Autodesk Fusion 360 part; units mm, degrees
(part 2 of 2)
  measures "d135" diameter of A4
extrude "Extrude12" add sketch "Lid (main and holes)" along normal blind 2 separate body makes body 2
extrude "Extrude13" add sketch "Lid (main and holes)" against normal blind 44 contours L2 L7 L8 L9 L12 L13 bodies 2
chamfer "Chamfer4" distance 2 angle 45 6 edges at (79.5, -47.5, 20) (79.5, 1, 42) (0, 49.5, 42) (-79.5, 1, 42) (-79.5, -47.5, 20) (0, -47.5, -2) on bodies 2
sketch "Lid (bottom holes)" plane through (0, -47.5, 0) normal (0, 1, 0) x (-1, 0, 0)
  line L0 (77.5, 0) -> (77.5, 42)
  line L1 (77.5, 42) -> (-77.5, 42)
  line L2 (-77.5, 42) -> (-77.5, 0)
  line L3 (-77.5, 0) -> (77.5, 0)
  line L4 (-75.5, 19) -> (-77.5, 19)
  line L5 (-77.5, 19) -> (-77.5, 23)
  line L6 (-77.5, 23) -> (-75.5, 23)
  line L7 (-75.5, 23) -> (-75.5, 19)
  line L8 (-75.5, 19) -> (-77.5, 23) construction
  line L9 (-77.5, 19) -> (-75.5, 23) construction
  line L10 (-2, 0) -> (2, 0)
  line L11 (2, 0) -> (2, 2)
  line L12 (2, 2) -> (-2, 2)
  line L13 (-2, 2) -> (-2, 0)
  line L14 (-2, 0) -> (2, 2) construction
  line L15 (2, 0) -> (-2, 2) construction
  line L16 (75.5, 19) -> (77.5, 19)
  line L17 (77.5, 19) -> (77.5, 23)
  line L18 (77.5, 23) -> (75.5, 23)
  line L19 (75.5, 23) -> (75.5, 19)
  line L20 (75.5, 19) -> (77.5, 23) construction
  line L21 (77.5, 19) -> (75.5, 23) construction
  point P0 (-76.5, 21)
  point P1 (-77.5, 21)
  point P2 (-77.5, 21)
  point P3 (0, 1)
  point P4 (77.5, 21)
  point P5 (76.5, 21)
  point P6 (77.5, 21)
  dimension "d82" = 2
  dimension "d83" = 4
  dimension "d84" = 4
  dimension "d85" = 2
  dimension "d86" = 2
  dimension "d87" = 4
  constraint horizontal L4
  constraint perpendicular L4 L5
  constraint parallel L4 L6
  constraint parallel L5 L7
  constraint coincident L8 P0
  constraint coincident L9 P0
  constraint midpoint L5 P2
  constraint midpoint L2 P2
  constraint coincident P2 P1
  constraint horizontal L10
  constraint perpendicular L10 L11
  constraint parallel L10 L12
  constraint parallel L11 L13
  constraint coincident L14 P3
  constraint coincident L15 P3
  constraint midpoint L0 P6
  constraint horizontal L16
  constraint perpendicular L16 L17
  constraint parallel L16 L18
  constraint parallel L17 L19
  constraint coincident L20 P5
  constraint coincident L21 P5
  constraint midpoint L17 P6
  constraint coincident P6 P4
  constraint midpoint L10 origin
  constraint midpoint L3 origin
  measures "d82" distance of L5.end L6.end
  measures "d83" distance of L4.end L5.end
  measures "d84" distance of L11.end L12.end
  measures "d85" distance of L10.end L11.end
  measures "d86" distance of L17.end L18.end
  measures "d87" distance of L16.end L17.end
extrude "Extrude14" cut sketch "Lid (bottom holes)" against normal up to surface (2 mm away) contours L0 L16 L17 L18 L19 | L3 L10 L11 L12 L13 | L2 L4 L5 L6 L7 bodies 2
sketch "Box (bolt spheres)" plane through (77.5, -2, 42) normal (0, 0, 1) x (1, 0, 0)
  arc A0 (-145, -45.5) -> (-155, -35.5) centre (-155, -45.5) ccw
  line L0 (-155, -45.5) -> (-155, 0)
  line L1 (-79.5, -45.5) -> (-155, -45.5)
  circle A1 centre (-150.8579, -41.3579) radius 1
  circle A2 centre (-150.8579, 45.3579) radius 1
  arc A3 (-155, 39.5) -> (-145, 49.5) centre (-155, 49.5) ccw
  line L2 (-155, 49.5) -> (-79.5, 49.5)
  line L3 (-155, 4) -> (-155, 49.5)
  circle A4 centre (-4.1421, 45.3579) radius 1
  arc A5 (-10, 49.5) -> (0, 39.5) centre (0, 49.5) ccw
  line L4 (-75.5, 49.5) -> (0, 49.5)
  line L5 (0, 49.5) -> (0, 4)
  circle A6 centre (-4.1421, -41.3579) radius 1
  arc A7 (0, -35.5) -> (-10, -45.5) centre (0, -45.5) ccw
  line L6 (0, 0) -> (0, -45.5)
  line L7 (0, -45.5) -> (-75.5, -45.5)
  point P0 (-155, -45.5)
  point P1 (-155, -45.5)
  point P2 (-140.8579, -45.5)
  point P3 (-150.8579, -41.3579)
  point P4 (-155, 49.5)
  point P5 (-155, 35.3579)
  point P6 (-155, 49.5)
  point P7 (-155, 49.5)
  point P8 (-150.8579, 45.3579)
  point P9 (-155, 49.5)
  point P10 (0, 49.5)
  point P11 (0, 49.5)
  point P12 (-4.1421, 45.3579)
  point P13 (0, 49.5)
  point P14 (-14.1421, 49.5)
  point P15 (0, 49.5)
  point P16 (0, -31.3579)
  point P17 (0, -45.5)
  point P18 (0, -45.5)
  point P19 (-4.1421, -41.3579)
  point P20 (0, -45.5)
  point P21 (0, -45.5)
  point P22 (0, -45.5)
  dimension "d90" = 10
  dimension "d92" = 14.1421
  dimension "d94" = 22.5
  dimension "d95" = 45
  dimension "d96" = 2
  dimension "d97" = 10
  dimension "d98" = 14.1421
  dimension "d99" = 22.5
  dimension "d100" = 45
  dimension "d101" = 2
  dimension "d102" = 10
  dimension "d103" = 14.1421
  dimension "d104" = 22.5
  dimension "d105" = 45
  dimension "d106" = 2
  dimension "d107" = 10
  dimension "d108" = 14.1421
  dimension "d109" = 22.5
  dimension "d110" = 45
  dimension "d111" = 2
  constraint coincident P0 A0.centre
  constraint coincident P1 P0
  constraint coincident A0.end L0
  constraint coincident A0.start L1
  constraint coincident L1 P2
  constraint coincident P3 A1.centre
  constraint coincident P9 P7
  constraint coincident P8 A2.centre
  constraint coincident A3.end L2
  constraint coincident A3.start L3
  constraint coincident P5 L3
  constraint coincident P15 P13
  constraint coincident P12 A4.centre
  constraint coincident A5.start L4
  constraint coincident P14 L4
  constraint coincident A5.end L5
  constraint coincident P22 P21
  constraint coincident P19 A6.centre
  constraint coincident A7.start L6
  constraint coincident A7.end L7
  constraint coincident P16 L6
  measures "d90" radius of A0
  measures "d92" distance of P0 P2
  measures "d94" angle of P1 P2 A1.centre
  measures "d95" angle of P1 P2 A1.centre
  measures "d96" diameter of A1
  measures "d97" radius of A3
  measures "d98" distance of P5 P9
  measures "d99" angle of P5 P8 P9
  measures "d100" angle of P5 P8 P9
  measures "d101" diameter of A2
  measures "d102" radius of A5
  measures "d103" distance of P14 P15
  measures "d104" angle of P12 P14 P15
  measures "d105" angle of P12 P14 P15
  measures "d106" diameter of A4
  measures "d107" radius of A7
  measures "d108" distance of P16 P22
  measures "d109" angle of P16 P19 P22
  measures "d110" angle of P16 P19 P22
  measures "d111" diameter of A6
revolve "Revolve2" add sketch "Box (bolt spheres)" angle 90 about axis through (77.5, 2, 42) along (0, -1, 0) contours A4 | A5 L4 L5 | A6 | A7 L6 L7 bodies 1
revolve "Revolve1" add sketch "Box (bolt spheres)" angle 90 about axis through (-77.5, -2, 42) along (0, 1, 0) contours A0 L0 L1 | A1 | A2 | A3 L2 L3 bodies 1
extrude "Extrude15" cut sketch "Box (bolt spheres)" against normal blind 10 contours A1 | A2 | A4 | A6 bodies 1
ref_plane "WorkPlane3" through (-77.5, -47.5, 23) normal (0, -1, 0) x (1, 0, 0)
sketch "Sketch8" plane through (-77.5, -47.5, 23) normal (0, -1, 0) x (1, 0, 0)
  line L0 (155, 19) -> (0, 19)
  line L1 (0, 19) -> (0, -23)
  line L2 (0, -23) -> (155, -23)
  line L3 (155, -23) -> (155, 19)
  line L4 (155, -23) -> (0, 19) construction
  line L5 (155, 19) -> (0, -23) construction
  line L6 (157, 21) -> (-2, 21) construction
  line L7 (-2, 21) -> (-2, -25) construction
  line L8 (-2, -25) -> (157, -25) construction
  line L9 (157, -25) -> (157, 21) construction
  line L10 (157, 21) -> (-2, -25) construction
  line L11 (-2, 21) -> (157, -25) construction
  point P0 (155, 19)
  point P1 (0, -23)
  point P2 (77.5, -2)
  point P3 (77.5, -2)
  dimension "d67" = 2
  dimension "d68" = 2
  constraint horizontal L0
  constraint vertical L1
  constraint horizontal L2
  constraint vertical L3
  constraint coincident P0 L0.start
  constraint coincident P1 L1.end
  constraint midpoint L5 P3
  constraint horizontal L6
  constraint perpendicular L6 L7
  constraint parallel L6 L8
  constraint parallel L7 L9
  constraint coincident L10 P3
  constraint coincident L11 P3
  constraint coincident P3 P2
  measures "d67" distance of L0 L6
  measures "d68" distance of L3 L9
ref_plane "WorkPlane2" through (-79.5, 49.5, 44) normal (0, 0, -1) x (-1, 0, 0)
sketch "Lid (main with holes)" plane through (-79.5, 49.5, 44) normal (0, 0, -1) x (1, 0, 0)
  line L0 (159, 99) -> (0, 99)
  line L1 (0, 99) -> (0, 0)
  line L2 (0, 0) -> (159, 0)
  line L3 (159, 0) -> (159, 99)
  line L4 (159, 99) -> (0, 99)
  line L5 (0, 99) -> (0, 97)
  line L6 (0, 97) -> (159, 97)
  line L7 (159, 97) -> (159, 99)
  spline S0 degree 3 poles (77.5984, 81.1332) (77.5984, 80.9632) (77.7282, 80.0784) (77.887, 79.1669) knots 0 0 0 0 1 1 1 1
  spline S1 degree 3 poles (77.887, 79.1669) (78.2333, 77.1783) (77.751, 75.0906) (76.6779, 73.9327) knots 0 0 0 0 1 1 1 1
  spline S2 degree 3 poles (76.6779, 73.9327) (76.311, 73.5368) (76.0109, 73.1615) (76.0109, 73.0987) knots 0 0 0 0 1 1 1 1
  spline S3 degree 3 poles (76.0109, 73.0987) (76.0109, 73.0359) (76.5764, 72.6966) (77.2676, 72.3448) knots 0 0 0 0 1 1 1 1
  spline S4 degree 3 poles (77.2676, 72.3448) (78.8144, 71.5575) (79.5559, 70.7799) (80.7771, 68.6645) knots 0 0 0 0 1 1 1 1
  line L8 (80.7771, 68.6645) -> (81.725, 67.0225)
  line L9 (81.725, 67.0225) -> (83.6966, 66.8902)
  line L10 (83.6966, 66.8902) -> (85.6682, 66.7579)
  line L11 (85.6682, 66.7579) -> (85.6197, 65.9642)
  spline S5 degree 3 poles (85.6197, 65.9642) (85.593, 65.5276) (85.4874, 64.5327) (85.3849, 63.7533) knots 0 0 0 0 1 1 1 1
  spline S6 degree 3 poles (85.3849, 63.7533) (85.2432, 62.6757) (85.2865, 62.2805) (85.5657, 62.1037) knots 0 0 0 0 1 1 1 1
  spline S7 degree 3 poles (85.5657, 62.1037) (86.2002, 61.7018) (87.0935, 61.8422) (87.3866, 62.3898) knots 0 0 0 0 1 1 1 1
  spline S8 degree 3 poles (87.3866, 62.3898) (87.8319, 63.2218) (87.7859, 64.7168) (87.2985, 65.2554) knots 0 0 0 0 1 1 1 1
  spline S9 degree 3 poles (87.2985, 65.2554) (86.7861, 65.8216) (86.7632, 66.1385) (87.1376, 67.4866) knots 0 0 0 0 1 1 1 1
  spline S10 degree 3 poles (87.1376, 67.4866) (87.3482, 68.2451) (87.6547, 68.603) (88.434, 69.0006) knots 0 0 0 0 1 1 1 1
  spline S11 degree 3 poles (88.434, 69.0006) (90.5941, 70.1026) (91.2091, 71.9528) (89.7692, 73.0174) knots 0 0 0 0 1 1 1 1
  spline S12 degree 3 poles (89.7692, 73.0174) (89.3326, 73.3402) (88.9755, 73.7045) (88.9755, 73.8271) knots 0 0 0 0 1 1 1 1
  spline S13 degree 3 poles (88.9755, 73.8271) (88.9755, 74.239) (91.9761, 77.596) (93.26, 78.6205) knots 0 0 0 0 1 1 1 1
  spline S14 degree 3 poles (93.26, 78.6205) (94.8501, 79.8892) (94.8873, 80.2345) (93.4072, 79.9864) knots 0 0 0 0 1 1 1 1
  spline S15 degree 3 poles (93.4072, 79.9864) (92.7888, 79.8828) (91.3357, 79.781) (90.1781, 79.7602) knots 0 0 0 0 1 1 1 1
  line L12 (90.1781, 79.7602) -> (88.0735, 79.7225)
  line L13 (88.0735, 79.7225) -> (87.8879, 78.8209)
  spline S16 degree 3 poles (87.8879, 78.8209) (87.6981, 77.8988) (87.3294, 77.5645) (85.9315, 77.0468) knots 0 0 0 0 1 1 1 1
  spline S17 degree 3 poles (85.9315, 77.0468) (84.7772, 76.6194) (84.1316, 76.9723) (82.7033, 78.8116) knots 0 0 0 0 1 1 1 1
  spline S18 degree 3 poles (82.7033, 78.8116) (82.0086, 79.706) (80.9974, 80.6639) (80.4559, 80.9401) knots 0 0 0 0 1 1 1 1
  spline S19 degree 3 poles (80.4559, 80.9401) (79.3609, 81.4987) (77.5984, 81.6178) (77.5984, 81.1332) knots 0 0 0 0 1 1 1 1
  spline S20 degree 3 poles (118.7262, 78.1114) (116.4189, 76.2321) (114.8749, 75.5697) (112.1171, 75.276) knots 0 0 0 0 1 1 1 1
  spline S21 degree 3 poles (112.1171, 75.276) (110.1488, 75.0664) (109.5837, 75.0907) (108.9721, 75.4111) knots 0 0 0 0 1 1 1 1
  spline S22 degree 3 poles (108.9721, 75.4111) (108.3328, 75.7461) (108.0142, 75.7518) (106.7369, 75.4512) knots 0 0 0 0 1 1 1 1
  spline S23 degree 3 poles (106.7369, 75.4512) (104.5652, 74.94) (104.145, 74.9973) (103.3311, 75.9155) knots 0 0 0 0 1 1 1 1
  spline S24 degree 3 poles (103.3311, 75.9155) (102.327, 77.0485) (101.6267, 77.2721) (100.5248, 76.8117) knots 0 0 0 0 1 1 1 1
  spline S25 degree 3 poles (100.5248, 76.8117) (99.8592, 76.5336) (99.3871, 76.5014) (98.7319, 76.6893) knots 0 0 0 0 1 1 1 1
  spline S26 degree 3 poles (98.7319, 76.6893) (97.5016, 77.0421) (97.5296, 77.0565) (97.3551, 75.9816) knots 0 0 0 0 1 1 1 1
  spline S27 degree 3 poles (97.3551, 75.9816) (97.2518, 75.3448) (97.3296, 74.8323) (97.5851, 74.4676) knots 0 0 0 0 1 1 1 1
  spline S28 degree 3 poles (97.5851, 74.4676) (97.7975, 74.1643) (97.9713, 73.4461) (97.9713, 72.8714) knots 0 0 0 0 1 1 1 1
  spline S29 degree 3 poles (97.9713, 72.8714) (97.9713, 72.2802) (98.1571, 71.6213) (98.3994, 71.3536) knots 0 0 0 0 1 1 1 1
  spline S30 degree 3 poles (98.3994, 71.3536) (98.6348, 71.0935) (98.9065, 70.4888) (99.0031, 70.0099) knots 0 0 0 0 1 1 1 1
  spline S31 degree 3 poles (99.0031, 70.0099) (99.1809, 69.1281) (100.0929, 68.4653) (102.7338, 67.2982) knots 0 0 0 0 1 1 1 1
  spline S32 degree 3 poles (102.7338, 67.2982) (103.2431, 67.0732) (104.2712, 66.5734) (105.0185, 66.1877) knots 0 0 0 0 1 1 1 1
  spline S33 degree 3 poles (105.0185, 66.1877) (106.2922, 65.5303) (106.4741, 65.5045) (107.9289, 65.7753) knots 0 0 0 0 1 1 1 1
  spline S34 degree 3 poles (107.9289, 65.7753) (108.7824, 65.9342) (110.6118, 66.2074) (111.9942, 66.3824) knots 0 0 0 0 1 1 1 1
  spline S35 degree 3 poles (111.9942, 66.3824) (114.7347, 66.7294) (115.0846, 66.854) (116.5529, 68.0048) knots 0 0 0 0 1 1 1 1
  spline S36 degree 3 poles (116.5529, 68.0048) (117.2007, 68.5126) (117.6345, 69.1302) (117.8156, 69.8027) knots 0 0 0 0 1 1 1 1
  spline S37 degree 3 poles (117.8156, 69.8027) (118.1252, 70.9524) (118.3828, 71.0819) (120.4609, 71.1329) knots 0 0 0 0 1 1 1 1
  spline S38 degree 3 poles (120.4609, 71.1329) (123.6168, 71.2104) (123.7034, 71.1882) (125.1383, 69.9329) knots 0 0 0 0 1 1 1 1
  spline S39 degree 3 poles (125.1383, 69.9329) (126.8725, 68.4159) (127.4525, 68.4114) (129.0987, 69.9017) knots 0 0 0 0 1 1 1 1
  spline S40 degree 3 poles (129.0987, 69.9017) (130.365, 71.0482) (130.3756, 71.0714) (130.0503, 71.971) knots 0 0 0 0 1 1 1 1
  spline S41 degree 3 poles (130.0503, 71.971) (129.8694, 72.4715) (129.7213, 73.0626) (129.7213, 73.2847) knots 0 0 0 0 1 1 1 1
  spline S42 degree 3 poles (129.7213, 73.2847) (129.7213, 73.6505) (131.8617, 75.7008) (132.8045, 76.2381) knots 0 0 0 0 1 1 1 1
  spline S43 degree 3 poles (132.8045, 76.2381) (133.2836, 76.5111) (132.9524, 76.9676) (131.7247, 77.7264) knots 0 0 0 0 1 1 1 1
  line L14 (131.7247, 77.7264) -> (130.8771, 78.2502)
  line L15 (130.8771, 78.2502) -> (129.0827, 77.6232)
  spline S44 degree 3 poles (129.0827, 77.6232) (127.6945, 77.1381) (127.0998, 77.0502) (126.456, 77.2349) knots 0 0 0 0 1 1 1 1
  spline S45 degree 3 poles (126.456, 77.2349) (125.9983, 77.3661) (125.1706, 77.4735) (124.6167, 77.4735) knots 0 0 0 0 1 1 1 1
  spline S46 degree 3 poles (124.6167, 77.4735) (123.5503, 77.4735) (122.3176, 77.9958) (121.4281, 78.8246) knots 0 0 0 0 1 1 1 1
  spline S47 degree 3 poles (121.4281, 78.8246) (120.6601, 79.5401) (120.394, 79.4699) (118.7262, 78.1114) knots 0 0 0 0 1 1 1 1
  spline S48 degree 3 poles (65.5754, 77.3267) (63.6541, 76.9083) (62.5009, 76.5165) (62.1461, 76.1618) knots 0 0 0 0 1 1 1 1
  spline S49 degree 3 poles (62.1461, 76.1618) (61.4175, 75.4332) (61.7596, 75.1794) (63.9385, 74.8323) knots 0 0 0 0 1 1 1 1
  spline S50 degree 3 poles (63.9385, 74.8323) (64.9385, 74.673) (66.4753, 74.2402) (67.3536, 73.8705) knots 0 0 0 0 1 1 1 1
  spline S51 degree 3 poles (67.3536, 73.8705) (68.79, 73.2659) (69.071, 73.2287) (70.1485, 73.5) knots 0 0 0 0 1 1 1 1
  spline S52 degree 3 poles (70.1485, 73.5) (70.8074, 73.6659) (72.1641, 73.7752) (73.1634, 73.7428) knots 0 0 0 0 1 1 1 1
  spline S53 degree 3 poles (73.1634, 73.7428) (75.1346, 73.6788) (75.5827, 73.9046) (75.8777, 75.1101) knots 0 0 0 0 1 1 1 1
  spline S54 degree 3 poles (75.8777, 75.1101) (76.0338, 75.7477) (75.929, 75.8346) (74.1709, 76.5243) knots 0 0 0 0 1 1 1 1
  spline S55 degree 3 poles (74.1709, 76.5243) (72.0028, 77.375) (69.7597, 78.005) (68.9994, 77.9768) knots 0 0 0 0 1 1 1 1
  spline S56 degree 3 poles (68.9994, 77.9768) (68.7084, 77.9661) (67.1676, 77.6735) (65.5754, 77.3267) knots 0 0 0 0 1 1 1 1
  spline S57 degree 3 poles (28.3193, 74.6051) (27.2891, 73.9841) (26.7486, 72.7185) (26.957, 71.4152) knots 0 0 0 0 1 1 1 1
  spline S58 degree 3 poles (26.957, 71.4152) (27.1572, 70.1635) (26.9583, 69.2046) (26.3782, 68.6245) knots 0 0 0 0 1 1 1 1
  spline S59 degree 3 poles (26.3782, 68.6245) (25.9955, 68.2418) (26.041, 68.1709) (26.8993, 67.8123) knots 0 0 0 0 1 1 1 1
  spline S60 degree 3 poles (26.8993, 67.8123) (27.4165, 67.5962) (28.3781, 67.4194) (29.036, 67.4194) knots 0 0 0 0 1 1 1 1
  spline S61 degree 3 poles (29.036, 67.4194) (30.0984, 67.4194) (30.3938, 67.5656) (31.6746, 68.7255) knots 0 0 0 0 1 1 1 1
  spline S62 degree 3 poles (31.6746, 68.7255) (33.0539, 69.9746) (34.3989, 70.5897) (35.7579, 70.5929) knots 0 0 0 0 1 1 1 1
  spline S63 degree 3 poles (35.7579, 70.5929) (36.3852, 70.5945) (36.9785, 70.1813) (39.5969, 67.9199) knots 0 0 0 0 1 1 1 1
  spline S64 degree 3 poles (39.5969, 67.9199) (40.9966, 66.7111) (42.3776, 66.1402) (45.9807, 65.281) knots 0 0 0 0 1 1 1 1
  spline S65 degree 3 poles (45.9807, 65.281) (46.7083, 65.1075) (47.8818, 64.8126) (48.5885, 64.6257) knots 0 0 0 0 1 1 1 1
  spline S66 degree 3 poles (48.5885, 64.6257) (49.7769, 64.3113) (50.0204, 64.3376) (51.8274, 64.9746) knots 0 0 0 0 1 1 1 1
  spline S67 degree 3 poles (51.8274, 64.9746) (53.7206, 65.642) (53.8474, 65.6526) (55.9111, 65.3175) knots 0 0 0 0 1 1 1 1
  spline S68 degree 3 poles (55.9111, 65.3175) (57.0825, 65.1273) (58.0746, 65.0163) (58.1157, 65.071) knots 0 0 0 0 1 1 1 1
  spline S69 degree 3 poles (58.1157, 65.071) (58.1569, 65.1257) (58.4591, 65.5592) (58.7872, 66.0343) knots 0 0 0 0 1 1 1 1
  spline S70 degree 3 poles (58.7872, 66.0343) (59.5311, 67.1114) (60.4072, 67.5691) (62.1864, 67.81) knots 0 0 0 0 1 1 1 1
  spline S71 degree 3 poles (62.1864, 67.81) (62.9504, 67.9135) (63.5755, 68.0925) (63.5755, 68.2078) knots 0 0 0 0 1 1 1 1
  spline S72 degree 3 poles (63.5755, 68.2078) (63.5755, 68.3231) (62.8718, 68.9326) (62.0117, 69.5623) knots 0 0 0 0 1 1 1 1
  spline S73 degree 3 poles (62.0117, 69.5623) (60.1594, 70.9184) (59.5482, 71.8233) (59.7621, 72.8928) knots 0 0 0 0 1 1 1 1
  spline S74 degree 3 poles (59.7621, 72.8928) (59.904, 73.6021) (59.8179, 73.7039) (58.5915, 74.2783) knots 0 0 0 0 1 1 1 1
  spline S75 degree 3 poles (58.5915, 74.2783) (57.2996, 74.8834) (57.2052, 74.89) (54.6669, 74.5514) knots 0 0 0 0 1 1 1 1
  spline S76 degree 3 poles (54.6669, 74.5514) (51.1868, 74.0872) (43.2934, 74.1772) (41.7981, 74.6981) knots 0 0 0 0 1 1 1 1
  spline S77 degree 3 poles (41.7981, 74.6981) (40.3198, 75.2132) (40.0364, 75.1928) (39.3204, 74.5202) knots 0 0 0 0 1 1 1 1
  spline S78 degree 3 poles (39.3204, 74.5202) (38.772, 74.005) (38.6094, 73.9787) (37.6852, 74.2556) knots 0 0 0 0 1 1 1 1
  spline S79 degree 3 poles (37.6852, 74.2556) (36.3353, 74.66) (35.284, 74.6308) (34.4713, 74.1662) knots 0 0 0 0 1 1 1 1
  spline S80 degree 3 poles (34.4713, 74.1662) (33.5031, 73.6128) (32.7139, 73.6859) (31.6177, 74.4308) knots 0 0 0 0 1 1 1 1
  spline S81 degree 3 poles (31.6177, 74.4308) (30.5061, 75.1862) (29.3819, 75.2456) (28.3193, 74.6051) knots 0 0 0 0 1 1 1 1
  spline S82 degree 3 poles (69.5947, 71.9995) (69.1174, 71.8747) (68.9423, 71.3881) (69.3747, 71.3881) knots 0 0 0 0 1 1 1 1
  spline S83 degree 3 poles (69.3747, 71.3881) (69.5084, 71.3881) (69.8676, 70.9838) (70.173, 70.4896) knots 0 0 0 0 1 1 1 1
  spline S84 degree 3 poles (70.173, 70.4896) (70.4959, 69.9672) (71.031, 69.5175) (71.4514, 69.4152) knots 0 0 0 0 1 1 1 1
  spline S85 degree 3 poles (71.4514, 69.4152) (72.7942, 69.0884) (74.1847, 67.9572) (74.7138, 66.7611) knots 0 0 0 0 1 1 1 1
  spline S86 degree 3 poles (74.7138, 66.7611) (75.3123, 65.4081) (76.8543, 64.5089) (78.5761, 64.5089) knots 0 0 0 0 1 1 1 1
  spline S87 degree 3 poles (78.5761, 64.5089) (79.4469, 64.5089) (79.9429, 64.2826) (81.1847, 63.3183) knots 0 0 0 0 1 1 1 1
  spline S88 degree 3 poles (81.1847, 63.3183) (82.028, 62.6635) (82.8078, 62.1277) (82.9175, 62.1277) knots 0 0 0 0 1 1 1 1
  spline S89 degree 3 poles (82.9175, 62.1277) (83.0273, 62.1277) (83.3057, 62.7765) (83.5362, 63.5694) knots 0 0 0 0 1 1 1 1
  spline S90 degree 3 poles (83.5362, 63.5694) (83.7667, 64.3624) (84.0728, 65.0838) (84.2164, 65.1725) knots 0 0 0 0 1 1 1 1
  spline S91 degree 3 poles (84.2164, 65.1725) (84.36, 65.2613) (84.4775, 65.4925) (84.4775, 65.6863) knots 0 0 0 0 1 1 1 1
  spline S92 degree 3 poles (84.4775, 65.6863) (84.4775, 65.9391) (83.9235, 66.0666) (82.5166, 66.1376) knots 0 0 0 0 1 1 1 1
  spline S93 degree 3 poles (82.5166, 66.1376) (80.2473, 66.2522) (79.8729, 66.4958) (78.6588, 68.647) knots 0 0 0 0 1 1 1 1
  spline S94 degree 3 poles (78.6588, 68.647) (77.7412, 70.2728) (76.6024, 71.3836) (75.3944, 71.831) knots 0 0 0 0 1 1 1 1
  spline S95 degree 3 poles (75.3944, 71.831) (74.5859, 72.1304) (70.5449, 72.2478) (69.5947, 71.9995) knots 0 0 0 0 1 1 1 1
  spline S96 degree 3 poles (62.1202, 64.2875) (61.0256, 63.6199) (59.7322, 62.0932) (58.9448, 60.5392) knots 0 0 0 0 1 1 1 1
  spline S97 degree 3 poles (58.9448, 60.5392) (57.9678, 58.6112) (58.0529, 58.112) (59.477, 57.4201) knots 0 0 0 0 1 1 1 1
  spline S98 degree 3 poles (59.477, 57.4201) (60.4925, 56.9267) (61.4722, 55.854) (61.8035, 54.8727) knots 0 0 0 0 1 1 1 1
  spline S99 degree 3 poles (61.8035, 54.8727) (61.8487, 54.7387) (62.7506, 54.5367) (63.8078, 54.4238) knots 0 0 0 0 1 1 1 1
  spline S100 degree 3 poles (63.8078, 54.4238) (65.1441, 54.281) (66.1012, 54.0008) (66.9486, 53.5042) knots 0 0 0 0 1 1 1 1
  spline S101 degree 3 poles (66.9486, 53.5042) (67.8563, 52.9722) (68.6449, 52.7569) (70.0386, 52.6606) knots 0 0 0 0 1 1 1 1
  spline S102 degree 3 poles (70.0386, 52.6606) (72.0894, 52.5189) (75.1036, 51.2477) (75.8225, 50.2212) knots 0 0 0 0 1 1 1 1
  spline S103 degree 3 poles (75.8225, 50.2212) (76.0618, 49.8795) (76.9257, 49.4801) (78.1572, 49.1417) knots 0 0 0 0 1 1 1 1
  spline S104 degree 3 poles (78.1572, 49.1417) (79.2323, 48.8462) (80.5708, 48.3036) (81.1316, 47.9358) knots 0 0 0 0 1 1 1 1
  spline S105 degree 3 poles (81.1316, 47.9358) (82.3787, 47.118) (84.2959, 46.8836) (86.4619, 47.2841) knots 0 0 0 0 1 1 1 1
  spline S106 degree 3 poles (86.4619, 47.2841) (88.2656, 47.6177) (89.2912, 48.258) (89.5096, 49.187) knots 0 0 0 0 1 1 1 1
  spline S107 degree 3 poles (89.5096, 49.187) (89.631, 49.7029) (90.1315, 50.0127) (92.1338, 50.8108) knots 0 0 0 0 1 1 1 1
  spline S108 degree 3 poles (92.1338, 50.8108) (93.4946, 51.3533) (94.6664, 51.8555) (94.7378, 51.9268) knots 0 0 0 0 1 1 1 1
  spline S109 degree 3 poles (94.7378, 51.9268) (94.8091, 51.9982) (94.7421, 52.3878) (94.5888, 52.7926) knots 0 0 0 0 1 1 1 1
  spline S110 degree 3 poles (94.5888, 52.7926) (94.4355, 53.1975) (94.239, 53.8547) (94.1521, 54.253) knots 0 0 0 0 1 1 1 1
  spline S111 degree 3 poles (94.1521, 54.253) (93.9589, 55.1385) (93.1549, 55.6967) (91.7536, 55.9182) knots 0 0 0 0 1 1 1 1
  spline S112 degree 3 poles (91.7536, 55.9182) (90.7792, 56.0722) (90.6582, 56.0223) (90.2287, 55.2895) knots 0 0 0 0 1 1 1 1
  spline S113 degree 3 poles (90.2287, 55.2895) (89.5921, 54.2034) (88.3449, 53.8194) (86.5419, 54.1543) knots 0 0 0 0 1 1 1 1
  spline S114 degree 3 poles (86.5419, 54.1543) (84.433, 54.546) (83.9231, 54.8108) (82.6468, 56.1775) knots 0 0 0 0 1 1 1 1
  spline S115 degree 3 poles (82.6468, 56.1775) (80.6597, 58.3055) (79.3477, 58.5635) (75.5626, 57.5708) knots 0 0 0 0 1 1 1 1
  line L16 (75.5626, 57.5708) -> (73.32, 56.9826)
  line L17 (73.32, 56.9826) -> (71.4243, 58.0056)
  spline S116 degree 3 poles (71.4243, 58.0056) (68.8296, 59.4059) (68.6025, 59.6373) (68.6025, 60.8807) knots 0 0 0 0 1 1 1 1
  spline S117 degree 3 poles (68.6025, 60.8807) (68.6025, 62.0942) (67.8523, 63.4598) (66.7571, 64.2396) knots 0 0 0 0 1 1 1 1
  spline S118 degree 3 poles (66.7571, 64.2396) (65.7586, 64.9506) (63.2501, 64.9765) (62.1202, 64.2875) knots 0 0 0 0 1 1 1 1
  spline S119 degree 3 poles (75.0194, 64.0336) (74.8191, 63.9022) (74.6216, 62.8612) (74.5168, 61.3849) knots 0 0 0 0 1 1 1 1
  line L18 (74.5168, 61.3849) -> (74.3441, 58.9527)
  line L19 (74.3441, 58.9527) -> (76.1176, 58.9527)
  spline S120 degree 3 poles (76.1176, 58.9527) (77.5648, 58.9527) (78.0669, 59.0722) (78.8472, 59.6024) knots 0 0 0 0 1 1 1 1
  spline S121 degree 3 poles (78.8472, 59.6024) (79.8246, 60.2666) (80.2442, 60.2682) (80.2442, 59.6078) knots 0 0 0 0 1 1 1 1
  spline S122 degree 3 poles (80.2442, 59.6078) (80.2442, 58.9963) (81.0804, 58.7469) (82.6688, 58.8845) knots 0 0 0 0 1 1 1 1
  spline S123 degree 3 poles (82.6688, 58.8845) (83.8126, 58.9837) (84.1964, 59.1255) (84.29, 59.4834) knots 0 0 0 0 1 1 1 1
  spline S124 degree 3 poles (84.29, 59.4834) (84.4803, 60.2111) (84.1403, 60.5342) (82.7414, 60.9552) knots 0 0 0 0 1 1 1 1
  spline S125 degree 3 poles (82.7414, 60.9552) (82.031, 61.169) (81.0891, 61.6928) (80.6485, 62.1192) knots 0 0 0 0 1 1 1 1
  spline S126 degree 3 poles (80.6485, 62.1192) (79.2951, 63.4286) (75.8721, 64.5928) (75.0194, 64.0336) knots 0 0 0 0 1 1 1 1
  spline S127 degree 3 poles (90.1661, 61.537) (87.1652, 61.2635) (85.7089, 60.8463) (85.5894, 60.2259) knots 0 0 0 0 1 1 1 1
  spline S128 degree 3 poles (85.5894, 60.2259) (85.526, 59.8967) (85.8181, 59.7573) (86.8759, 59.6118) knots 0 0 0 0 1 1 1 1
  spline S129 degree 3 poles (86.8759, 59.6118) (89.1162, 59.3037) (92.636, 57.3719) (94.3703, 55.4987) knots 0 0 0 0 1 1 1 1
  spline S130 degree 3 poles (94.3703, 55.4987) (95.1848, 54.619) (95.9292, 53.5777) (96.0245, 53.1848) knots 0 0 0 0 1 1 1 1
  spline S131 degree 3 poles (96.0245, 53.1848) (96.3299, 51.926) (97.4458, 49.5707) (97.8985, 49.2293) knots 0 0 0 0 1 1 1 1
  spline S132 degree 3 poles (97.8985, 49.2293) (98.3548, 48.8851) (100.2652, 48.7801) (100.9924, 49.0591) knots 0 0 0 0 1 1 1 1
  spline S133 degree 3 poles (100.9924, 49.0591) (101.2225, 49.1474) (101.4109, 49.4901) (101.4109, 49.8205) knots 0 0 0 0 1 1 1 1
  spline S134 degree 3 poles (101.4109, 49.8205) (101.4109, 50.5308) (101.8033, 50.9044) (102.8166, 51.1587) knots 0 0 0 0 1 1 1 1
  spline S135 degree 3 poles (102.8166, 51.1587) (103.9802, 51.4507) (104.2985, 52.2013) (104.1816, 54.3772) knots 0 0 0 0 1 1 1 1
  spline S136 degree 3 poles (104.1816, 54.3772) (104.0195, 57.3929) (103.0669, 58.7882) (100.1803, 60.2374) knots 0 0 0 0 1 1 1 1
  spline S137 degree 3 poles (100.1803, 60.2374) (98.9744, 60.8428) (94.5549, 61.888) (93.4858, 61.8206) knots 0 0 0 0 1 1 1 1
  spline S138 degree 3 poles (93.4858, 61.8206) (93.1151, 61.7973) (91.6213, 61.6696) (90.1661, 61.537) knots 0 0 0 0 1 1 1 1
  spline S139 degree 3 poles (52.8787, 56.6848) (52.1441, 55.9502) (52.339, 53.9389) (53.2829, 52.5138) knots 0 0 0 0 1 1 1 1
  spline S140 degree 3 poles (53.2829, 52.5138) (56.0025, 48.408) (62.5608, 45.6251) (66.3312, 46.977) knots 0 0 0 0 1 1 1 1
  spline S141 degree 3 poles (66.3312, 46.977) (67.9586, 47.5605) (68.3705, 48.1317) (67.6989, 48.8737) knots 0 0 0 0 1 1 1 1
  spline S142 degree 3 poles (67.6989, 48.8737) (67.208, 49.4162) (64.9024, 50.2214) (63.8402, 50.2214) knots 0 0 0 0 1 1 1 1
  spline S143 degree 3 poles (63.8402, 50.2214) (62.4545, 50.2214) (61.2392, 51.7301) (60.2922, 54.6261) knots 0 0 0 0 1 1 1 1
  spline S144 degree 3 poles (60.2922, 54.6261) (59.7425, 56.3068) (58.8005, 56.8959) (57.2276, 56.5425) knots 0 0 0 0 1 1 1 1
  spline S145 degree 3 poles (57.2276, 56.5425) (56.5232, 56.3842) (55.8344, 56.4332) (54.937, 56.7055) knots 0 0 0 0 1 1 1 1
  spline S146 degree 3 poles (54.937, 56.7055) (53.3456, 57.1883) (53.3826, 57.1887) (52.8787, 56.6848) knots 0 0 0 0 1 1 1 1
  spline S147 degree 3 poles (105.4269, 53.8503) (105.2718, 53.6634) (105.1084, 52.8002) (105.0638, 51.9321) knots 0 0 0 0 1 1 1 1
  line L20 (105.0638, 51.9321) -> (104.9827, 50.3537)
  line L21 (104.9827, 50.3537) -> (103.4777, 50.2749)
  spline S148 degree 3 poles (103.4777, 50.2749) (102.0203, 50.1985) (101.9631, 50.167) (101.6706, 49.2806) knots 0 0 0 0 1 1 1 1
  spline S149 degree 3 poles (101.6706, 49.2806) (101.2976, 48.1504) (100.625, 47.7651) (99.4199, 47.9912) knots 0 0 0 0 1 1 1 1
  spline S150 degree 3 poles (99.4199, 47.9912) (98.1653, 48.2265) (97.7067, 47.7926) (97.7067, 46.3698) knots 0 0 0 0 1 1 1 1
  spline S151 degree 3 poles (97.7067, 46.3698) (97.7067, 44.7231) (97.316, 43.9289) (96.2575, 43.4241) knots 0 0 0 0 1 1 1 1
  spline S152 degree 3 poles (96.2575, 43.4241) (95.5257, 43.0752) (95.3255, 42.8238) (95.3255, 42.2538) knots 0 0 0 0 1 1 1 1
  spline S153 degree 3 poles (95.3255, 42.2538) (95.3255, 41.8546) (95.5108, 41.3426) (95.7374, 41.116) knots 0 0 0 0 1 1 1 1
  spline S154 degree 3 poles (95.7374, 41.116) (96.0958, 40.7576) (96.2249, 40.7525) (96.7296, 41.0768) knots 0 0 0 0 1 1 1 1
  spline S155 degree 3 poles (96.7296, 41.0768) (97.3866, 41.4989) (99.9696, 42.0194) (101.4077, 42.0194) knots 0 0 0 0 1 1 1 1
  spline S156 degree 3 poles (101.4077, 42.0194) (102.652, 42.0194) (104.2046, 43.0193) (106.5842, 45.3532) knots 0 0 0 0 1 1 1 1
  spline S157 degree 3 poles (106.5842, 45.3532) (108.8069, 47.5334) (109.3378, 48.824) (108.8135, 50.7727) knots 0 0 0 0 1 1 1 1
  spline S158 degree 3 poles (108.8135, 50.7727) (108.2139, 53.0015) (107.3463, 54.1902) (106.3192, 54.1902) knots 0 0 0 0 1 1 1 1
  spline S159 degree 3 poles (106.3192, 54.1902) (105.9836, 54.1902) (105.5821, 54.0372) (105.4269, 53.8503) knots 0 0 0 0 1 1 1 1
  spline S160 degree 3 poles (64.1251, 52.7596) (63.5162, 52.026) (64.0142, 51.6181) (66.5508, 50.773) knots 0 0 0 0 1 1 1 1
  spline S161 degree 3 poles (66.5508, 50.773) (68.8283, 50.0143) (69.1605, 49.8127) (70.5384, 48.3527) knots 0 0 0 0 1 1 1 1
  spline S162 degree 3 poles (70.5384, 48.3527) (71.6046, 47.2229) (72.5414, 46.5357) (73.7616, 45.9883) knots 0 0 0 0 1 1 1 1
  line L22 (73.7616, 45.9883) -> (75.4817, 45.2165)
  line L23 (75.4817, 45.2165) -> (75.4817, 44.0241)
  spline S163 degree 3 poles (75.4817, 44.0241) (75.4817, 42.3441) (75.8367, 42.2135) (80.1014, 42.3248) knots 0 0 0 0 1 1 1 1
  spline S164 degree 3 poles (80.1014, 42.3248) (82.7203, 42.3932) (83.7238, 42.5163) (84.0812, 42.8131) knots 0 0 0 0 1 1 1 1
  spline S165 degree 3 poles (84.0812, 42.8131) (84.4624, 43.1297) (85.4212, 43.21) (88.8178, 43.21) knots 0 0 0 0 1 1 1 1
  spline S166 degree 3 poles (88.8178, 43.21) (92.911, 43.21) (93.1331, 43.2378) (94.5338, 43.9257) knots 0 0 0 0 1 1 1 1
  spline S167 degree 3 poles (94.5338, 43.9257) (95.3896, 44.346) (96.1813, 44.9635) (96.452, 45.4217) knots 0 0 0 0 1 1 1 1
  spline S168 degree 3 poles (96.452, 45.4217) (97.0937, 46.5079) (97.0482, 47.9695) (96.3511, 48.6666) knots 0 0 0 0 1 1 1 1
  spline S169 degree 3 poles (96.3511, 48.6666) (95.8533, 49.1645) (95.5686, 49.2143) (93.8533, 49.1043) knots 0 0 0 0 1 1 1 1
  spline S170 degree 3 poles (93.8533, 49.1043) (91.6176, 48.9608) (90.6174, 48.4434) (90.3915, 47.3134) knots 0 0 0 0 1 1 1 1
  spline S171 degree 3 poles (90.3915, 47.3134) (90.223, 46.4713) (90.1313, 46.4358) (86.9911, 45.9943) knots 0 0 0 0 1 1 1 1
  spline S172 degree 3 poles (86.9911, 45.9943) (84.1582, 45.5961) (81.6682, 45.6589) (80.6941, 46.1531) knots 0 0 0 0 1 1 1 1
  spline S173 degree 3 poles (80.6941, 46.1531) (80.2284, 46.3893) (79.278, 46.9871) (78.5823, 47.4815) knots 0 0 0 0 1 1 1 1
  spline S174 degree 3 poles (78.5823, 47.4815) (77.8865, 47.9759) (76.6633, 48.5507) (75.864, 48.7589) knots 0 0 0 0 1 1 1 1
  spline S175 degree 3 poles (75.864, 48.7589) (74.8651, 49.0191) (74.2026, 49.3849) (73.7447, 49.9291) knots 0 0 0 0 1 1 1 1
  spline S176 degree 3 poles (73.7447, 49.9291) (73.0112, 50.8007) (70.6608, 51.804) (69.3202, 51.8176) knots 0 0 0 0 1 1 1 1
  spline S177 degree 3 poles (69.3202, 51.8176) (68.8527, 51.8223) (67.8154, 52.068) (67.015, 52.3635) knots 0 0 0 0 1 1 1 1
  spline S178 degree 3 poles (67.015, 52.3635) (64.8243, 53.1724) (64.5041, 53.2163) (64.1251, 52.7596) knots 0 0 0 0 1 1 1 1
  spline S179 degree 3 poles (53.2567, 49.8188) (53.2567, 49.7428) (53.6071, 48.9078) (54.0355, 47.9632) knots 0 0 0 0 1 1 1 1
  spline S180 degree 3 poles (54.0355, 47.9632) (54.5801, 46.7619) (55.2959, 45.7873) (56.4167, 44.7208) knots 0 0 0 0 1 1 1 1
  line L24 (56.4167, 44.7208) -> (58.0192, 43.1959)
  line L25 (58.0192, 43.1959) -> (58.0192, 41.2539)
  line L26 (58.0192, 41.2539) -> (58.0192, 39.3118)
  line L27 (58.0192, 39.3118) -> (58.7468, 39.5303)
  spline S181 degree 3 poles (58.7468, 39.5303) (59.147, 39.6505) (60.9032, 39.7367) (62.6494, 39.7217) knots 0 0 0 0 1 1 1 1
  spline S182 degree 3 poles (62.6494, 39.7217) (66.1489, 39.6918) (71.5047, 38.7078) (75.1914, 37.4173) knots 0 0 0 0 1 1 1 1
  spline S183 degree 3 poles (75.1914, 37.4173) (77.6172, 36.5682) (81.4416, 34.5419) (84.0788, 32.7084) knots 0 0 0 0 1 1 1 1
  spline S184 degree 3 poles (84.0788, 32.7084) (86.0375, 31.3468) (86.1121, 31.3203) (88.1202, 31.2746) knots 0 0 0 0 1 1 1 1
  spline S185 degree 3 poles (88.1202, 31.2746) (89.5903, 31.2412) (90.6717, 31.0362) (91.9627, 30.5461) knots 0 0 0 0 1 1 1 1
  spline S186 degree 3 poles (91.9627, 30.5461) (93.6114, 29.9203) (93.9163, 29.885) (95.6668, 30.1166) knots 0 0 0 0 1 1 1 1
  spline S187 degree 3 poles (95.6668, 30.1166) (97.6139, 30.3743) (101.1023, 31.3906) (102.4741, 32.1) knots 0 0 0 0 1 1 1 1
  spline S188 degree 3 poles (102.4741, 32.1) (102.8935, 32.3169) (103.451, 32.4962) (103.7128, 32.4984) knots 0 0 0 0 1 1 1 1
  spline S189 degree 3 poles (103.7128, 32.4984) (103.9747, 32.5006) (104.3676, 32.6154) (104.5859, 32.7534) knots 0 0 0 0 1 1 1 1
  spline S190 degree 3 poles (104.5859, 32.7534) (105.2189, 33.1537) (104.3508, 33.8287) (102.9686, 34.0109) knots 0 0 0 0 1 1 1 1
  spline S191 degree 3 poles (102.9686, 34.0109) (102.3301, 34.0951) (101.4393, 34.4432) (100.989, 34.7844) knots 0 0 0 0 1 1 1 1
  spline S192 degree 3 poles (100.989, 34.7844) (100.0356, 35.5069) (98.8173, 35.5822) (97.6713, 34.9896) knots 0 0 0 0 1 1 1 1
  spline S193 degree 3 poles (97.6713, 34.9896) (96.5305, 34.3996) (95.7579, 34.4447) (93.2225, 35.2492) knots 0 0 0 0 1 1 1 1
  spline S194 degree 3 poles (93.2225, 35.2492) (90.1177, 36.2343) (88.9615, 36.3563) (87.6607, 35.8358) knots 0 0 0 0 1 1 1 1
  spline S195 degree 3 poles (87.6607, 35.8358) (85.9885, 35.1667) (85.4736, 35.289) (83.5124, 36.8209) knots 0 0 0 0 1 1 1 1
  spline S196 degree 3 poles (83.5124, 36.8209) (80.8847, 38.8734) (80.2215, 39.1601) (78.3311, 39.0609) knots 0 0 0 0 1 1 1 1
  spline S197 degree 3 poles (78.3311, 39.0609) (76.0392, 38.9406) (75.958, 39.5337) (78.233, 39.7773) knots 0 0 0 0 1 1 1 1
  spline S198 degree 3 poles (78.233, 39.7773) (80.2684, 39.9953) (82.9286, 39.3145) (84.6295, 38.1403) knots 0 0 0 0 1 1 1 1
  spline S199 degree 3 poles (84.6295, 38.1403) (85.5652, 37.4943) (85.9172, 37.4191) (88.1817, 37.3812) knots 0 0 0 0 1 1 1 1
  spline S200 degree 3 poles (88.1817, 37.3812) (90.2012, 37.3474) (91.0524, 37.2011) (92.5127, 36.6366) knots 0 0 0 0 1 1 1 1
  spline S201 degree 3 poles (92.5127, 36.6366) (95.015, 35.6692) (96.6186, 35.6923) (98.0603, 36.7165) knots 0 0 0 0 1 1 1 1
  spline S202 degree 3 poles (98.0603, 36.7165) (98.9816, 37.3711) (99.5051, 37.5248) (101.259, 37.6557) knots 0 0 0 0 1 1 1 1
  spline S203 degree 3 poles (101.259, 37.6557) (102.4124, 37.7419) (103.4542, 37.873) (103.5741, 37.9471) knots 0 0 0 0 1 1 1 1
  spline S204 degree 3 poles (103.5741, 37.9471) (103.694, 38.0212) (103.7921, 38.6078) (103.7921, 39.2507) knots 0 0 0 0 1 1 1 1
  spline S205 degree 3 poles (103.7921, 39.2507) (103.7921, 40.1739) (103.667, 40.4996) (103.1968, 40.7998) knots 0 0 0 0 1 1 1 1
  spline S206 degree 3 poles (103.1968, 40.7998) (102.6737, 41.1339) (102.2968, 41.1196) (100.088, 40.6816) knots 0 0 0 0 1 1 1 1
  spline S207 degree 3 poles (100.088, 40.6816) (96.2725, 39.9251) (95.7598, 39.9723) (94.8905, 41.1595) knots 0 0 0 0 1 1 1 1
  spline S208 degree 3 poles (94.8905, 41.1595) (94.4909, 41.7052) (94.0809, 42.252) (93.9793, 42.3747) knots 0 0 0 0 1 1 1 1
  spline S209 degree 3 poles (93.9793, 42.3747) (93.8777, 42.4974) (93.4859, 42.3956) (93.1087, 42.1484) knots 0 0 0 0 1 1 1 1
  spline S210 degree 3 poles (93.1087, 42.1484) (92.5137, 41.7586) (92.2006, 41.7378) (90.7437, 41.9915) knots 0 0 0 0 1 1 1 1
  spline S211 degree 3 poles (90.7437, 41.9915) (88.1701, 42.4397) (86.4733, 42.3637) (85.4761, 41.7558) knots 0 0 0 0 1 1 1 1
  spline S212 degree 3 poles (85.4761, 41.7558) (84.9499, 41.4349) (84.1425, 41.2273) (83.4192, 41.227) knots 0 0 0 0 1 1 1 1
  spline S213 degree 3 poles (83.4192, 41.227) (82.7644, 41.2266) (80.9431, 41.0871) (79.3721, 40.9169) knots 0 0 0 0 1 1 1 1
  spline S214 degree 3 poles (79.3721, 40.9169) (76.0798, 40.5603) (76.2604, 40.4774) (74.951, 42.9454) knots 0 0 0 0 1 1 1 1
  spline S215 degree 3 poles (74.951, 42.9454) (73.1728, 46.2969) (71.4711, 47.1082) (68.4702, 46.0352) knots 0 0 0 0 1 1 1 1
  spline S216 degree 3 poles (68.4702, 46.0352) (67.0194, 45.5164) (62.3286, 44.8499) (61.1967, 45.0017) knots 0 0 0 0 1 1 1 1
  spline S217 degree 3 poles (61.1967, 45.0017) (59.9458, 45.1695) (56.3861, 47.4198) (54.8584, 49.0086) knots 0 0 0 0 1 1 1 1
  spline S218 degree 3 poles (54.8584, 49.0086) (54.0647, 49.8341) (53.2567, 50.2428) (53.2567, 49.8188) knots 0 0 0 0 1 1 1 1
  spline S219 degree 3 poles (60.7312, 37.918) (60.1372, 37.4924) (59.929, 36.2516) (60.2927, 35.3039) knots 0 0 0 0 1 1 1 1
  spline S220 degree 3 poles (60.2927, 35.3039) (60.4799, 34.816) (63.9271, 33.4446) (66.4231, 32.865) knots 0 0 0 0 1 1 1 1
  spline S221 degree 3 poles (66.4231, 32.865) (67.5786, 32.5966) (68.6902, 32.5113) (69.583, 32.6225) knots 0 0 0 0 1 1 1 1
  spline S222 degree 3 poles (69.583, 32.6225) (70.6653, 32.7573) (71.2235, 32.6777) (72.1889, 32.2506) knots 0 0 0 0 1 1 1 1
  spline S223 degree 3 poles (72.1889, 32.2506) (73.7125, 31.5767) (75.7519, 30.1015) (77.3916, 28.4872) knots 0 0 0 0 1 1 1 1
  spline S224 degree 3 poles (77.3916, 28.4872) (78.7159, 27.1834) (80.4547, 26.4089) (82.0574, 26.4089) knots 0 0 0 0 1 1 1 1
  spline S225 degree 3 poles (82.0574, 26.4089) (82.5662, 26.4089) (83.8646, 26.7134) (84.9426, 27.0855) knots 0 0 0 0 1 1 1 1
  spline S226 degree 3 poles (84.9426, 27.0855) (87.5605, 27.989) (89.2375, 28.1741) (90.2039, 27.6661) knots 0 0 0 0 1 1 1 1
  spline S227 degree 3 poles (90.2039, 27.6661) (90.6197, 27.4475) (91.3738, 27.053) (91.8798, 26.7895) knots 0 0 0 0 1 1 1 1
  spline S228 degree 3 poles (91.8798, 26.7895) (93.1515, 26.1271) (95.3032, 25.9808) (96.2744, 26.4908) knots 0 0 0 0 1 1 1 1
  spline S229 degree 3 poles (96.2744, 26.4908) (97.4166, 27.0907) (99.3924, 29.211) (99.1599, 29.5873) knots 0 0 0 0 1 1 1 1
  spline S230 degree 3 poles (99.1599, 29.5873) (99.0179, 29.817) (98.4075, 29.8518) (96.9462, 29.7133) knots 0 0 0 0 1 1 1 1
  spline S231 degree 3 poles (96.9462, 29.7133) (94.0883, 29.4424) (92.6457, 29.5119) (91.2435, 29.988) knots 0 0 0 0 1 1 1 1
  spline S232 degree 3 poles (91.2435, 29.988) (90.3739, 30.2832) (89.5778, 30.3524) (88.4797, 30.2281) knots 0 0 0 0 1 1 1 1
  spline S233 degree 3 poles (88.4797, 30.2281) (86.6583, 30.0221) (85.6819, 30.3817) (82.4546, 32.4474) knots 0 0 0 0 1 1 1 1
  spline S234 degree 3 poles (82.4546, 32.4474) (80.2109, 33.8836) (79.0405, 34.4003) (74.5557, 35.9345) knots 0 0 0 0 1 1 1 1
  spline S235 degree 3 poles (74.5557, 35.9345) (71.2653, 37.0601) (69.8113, 37.3863) (66.2213, 37.8043) knots 0 0 0 0 1 1 1 1
  spline S236 degree 3 poles (66.2213, 37.8043) (61.3907, 38.3667) (61.3585, 38.3674) (60.7312, 37.918) knots 0 0 0 0 1 1 1 1
  spline S237 degree 3 poles (67.4119, 29.993) (65.581, 29.6092) (64.8984, 29.352) (64.8984, 29.046) knots 0 0 0 0 1 1 1 1
  spline S238 degree 3 poles (64.8984, 29.046) (64.8984, 28.8092) (70.3204, 25.8321) (76.8605, 22.4779) knots 0 0 0 0 1 1 1 1
  line L28 (76.8605, 22.4779) -> (81.0174, 20.346)
  line L29 (81.0174, 20.346) -> (82.3986, 20.7561)
  spline S239 degree 3 poles (82.3986, 20.7561) (83.3465, 21.0376) (84.2248, 21.1107) (85.1988, 20.989) knots 0 0 0 0 1 1 1 1
  spline S240 degree 3 poles (85.1988, 20.989) (86.3664, 20.8431) (86.8122, 20.9129) (87.7138, 21.3828) knots 0 0 0 0 1 1 1 1
  spline S241 degree 3 poles (87.7138, 21.3828) (88.5671, 21.8276) (89.1648, 21.9346) (90.4139, 21.8664) knots 0 0 0 0 1 1 1 1
  spline S242 degree 3 poles (90.4139, 21.8664) (91.8929, 21.7856) (92.0246, 21.8238) (92.1003, 22.3557) knots 0 0 0 0 1 1 1 1
  spline S243 degree 3 poles (92.1003, 22.3557) (92.1643, 22.8052) (91.7533, 23.2557) (90.2401, 24.3946) knots 0 0 0 0 1 1 1 1
  spline S244 degree 3 poles (90.2401, 24.3946) (87.3666, 26.5574) (87.0773, 26.643) (84.0087, 26.2383) knots 0 0 0 0 1 1 1 1
  spline S245 degree 3 poles (84.0087, 26.2383) (78.8315, 25.5555) (78.1108, 25.7112) (74.0398, 28.3921) knots 0 0 0 0 1 1 1 1
  spline S246 degree 3 poles (74.0398, 28.3921) (70.8842, 30.4703) (70.3285, 30.6045) (67.4119, 29.993) knots 0 0 0 0 1 1 1 1
  spline S247 degree 3 poles (72.7697, 22.6836) (72.0539, 22.2667) (72.2209, 21.7073) (73.1201, 21.5098) knots 0 0 0 0 1 1 1 1
  spline S248 degree 3 poles (73.1201, 21.5098) (73.5675, 21.4116) (74.3326, 20.9808) (74.8204, 20.5525) knots 0 0 0 0 1 1 1 1
  spline S249 degree 3 poles (74.8204, 20.5525) (75.4668, 19.9849) (76.412, 19.5945) (78.3065, 19.1124) knots 0 0 0 0 1 1 1 1
  spline S250 degree 3 poles (78.3065, 19.1124) (81.238, 18.3666) (82.7056, 18.3518) (82.8411, 19.0668) knots 0 0 0 0 1 1 1 1
  spline S251 degree 3 poles (82.8411, 19.0668) (82.9157, 19.4606) (82.7183, 19.53) (81.5204, 19.5315) knots 0 0 0 0 1 1 1 1
  spline S252 degree 3 poles (81.5204, 19.5315) (80.5495, 19.5327) (79.8653, 19.6989) (79.3182, 20.0665) knots 0 0 0 0 1 1 1 1
  spline S253 degree 3 poles (79.3182, 20.0665) (78.4877, 20.6245) (73.6783, 22.9753) (73.3958, 22.9613) knots 0 0 0 0 1 1 1 1
  spline S254 degree 3 poles (73.3958, 22.9613) (73.3061, 22.9569) (73.0244, 22.8319) (72.7697, 22.6836) knots 0 0 0 0 1 1 1 1
  point P0 (159, 99)
  dimension "d59" = 2
  constraint horizontal L0
  constraint vertical L1
  constraint horizontal L2
  constraint vertical L3
  constraint coincident L1.end L2.start
  constraint coincident P0 L0.start
  constraint horizontal L4
  constraint vertical L5
  constraint horizontal L6
  constraint vertical L7
  constraint coincident L1 L5.end
  measures "d59" distance of L0 L6
extrude "Extrude9" [suppressed]
extrude "Extrude10" [suppressed]
chamfer "Chamfer3" [suppressed]
extrude "Extrude11" [suppressed]
chamfer "Chamfer1" [suppressed]
sketch "Sketch1" plane through (0, 0, 0) normal (1, 0, 0) x (0, 0, -1)
equation "d8 = d7"
equation "d9 = -d7"
equation "d11 = d16 + d23 + d26 + d16 + d27 + d7"
equation "d13 = d7"
equation "d14 = d7"
equation "d29 = d6"
equation "d36 = d31"
equation "d37 = d32"
equation "d40 = d7"
equation "d41 = d7"
equation "d42 = d32"
equation "d43 = d31"
equation "d44 = d31"
equation "d45 = d32"
equation "d55 = d5 / 4"
equation "d59 = d7"
equation "d60 = d7"
equation "d62 = d7 + d23 + d16 + d26 + d16 + d27 + d7"
equation "d64 = d7"
equation "d69 = d7"
equation "d71 = -( d23 + d16 + d26 + d16 + d27 + d7 )"
equation "d73 = d7"
equation "d74 = d31"
equation "d75 = d32"
equation "d78 = d32"
equation "d79 = d31"
equation "d80 = d32"
equation "d81 = d31"
equation "d82 = d32"
equation "d83 = d31"
equation "d84 = d31"
equation "d85 = d32"
equation "d86 = d32"
equation "d87 = d31"
equation "d92 = d90 * sqrt(2)"
equation "d97 = d90"
equation "d98 = d90 * sqrt(2)"
equation "d101 = d96"
equation "d102 = d90"
equation "d103 = d90 * sqrt(2)"
equation "d106 = d96"
equation "d107 = d90"
equation "d108 = d90 * sqrt(2)"
equation "d111 = d96"
equation "d114 = -d90"
equation "d117 = sqrt(2) * d90"
equation "d118 = d96"
equation "d121 = d96"
equation "d123 = sqrt(2) * d90"
equation "d127 = d96"
equation "d128 = sqrt(2) * d90"
equation "d131 = d96"
equation "d132 = sqrt(2) * d90"
equation "d135 = d96"
named bodies: "Box", "Lid"
